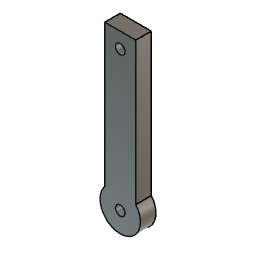
final Assembly (Autodesk Fusion 360 archive; units mm, degrees)
design "link"
Autodesk Fusion 360 part; units mm, degrees
sketch "Sketch1" plane through (0, 0, 0) normal (0, 1, 0) x (1, 0, 0)
  line L0 (0, 0) -> (10, 0)
  line L1 (10, 0) -> (10, 45.8467)
  line L2 (0, 45.8467) -> (0, 0)
  line L3 (0, 0) -> (5, 0)
  circle A0 centre (5, 5) radius 1.55
  circle A1 centre (5, 50) radius 1.55
  arc A2 (10, 45.8467) -> (0, 45.8467) centre (5, 50) ccw
  dimension "d1" = 10
  dimension "d4" = 3.1
  dimension "d5" = 3.1
  dimension "d6" = 13
  constraint horizontal L0
  constraint vertical L1
  constraint vertical L2
  constraint coincident L0.start L2.end
  constraint midpoint L0 L3.end
  constraint concentric A1 A2
  measures "d1" distance of L0.start L0.end
  measures "d4" diameter of A0
  measures "d5" diameter of A1
  measures "d6" diameter of A2
extrude "Extrude1" add sketch "Sketch1" along normal blind 5 contours L0 L1 L2 L3 A2 | A0
extrude "Extrude2" add sketch "Sketch1" along normal blind 10 contours L0 L1 L2 L3 A2 | A0
extrude "Extrude3" add sketch "Sketch1" against normal blind 3 contours L0 L1 L2 L3 A2 | A0
extrude "Extrude4" cut 1 faces at (6.6667, 10, -15.2822) along direction (0, -1, 0) blind 2
extrude "Extrude5" add sketch "Sketch1" against normal blind 8 contours A0
delete_face "DeleteFace1" 1 faces at (6.5423, -4.6667, -4.8457)
sketch "Sketch2" plane through (0, 0, 0) normal (0, 1, 0) x (1, 0, 0)
extrude "Extrude7" cut 1 faces at (6.6667, -3, -15.2822) along direction (0, 1, 0) blind 3
extrude "Extrude8" cut sketch "Sketch1" along normal blind 100 contours A0
extrude "Extrude9" cut 1 faces at (5.0386, 0, -32.7463) along direction (0, 1, 0) blind 3
sketch "Sketch3" plane through (0, 3, 0) normal (0, -1, 0) x (1, 0, 0)
  circle A0 centre (5, -5) radius 1.55
  circle A1 centre (5, -50) radius 1.55
  arc A2 (0, -45.8467) -> (10, -45.8467) centre (5, -50) ccw
  line L0 (10, -45.8467) -> (10, 0)
  line L1 (10, 0) -> (0, 0)
  line L2 (0, 0) -> (0, -45.8467)
extrude "Extrude6" [rolled back] along distance 5 taper angle 0
component "Component" placed x (1, 0, 0) y (0, 1, 0) z (0, 0, 1) at (0, 0, 0)

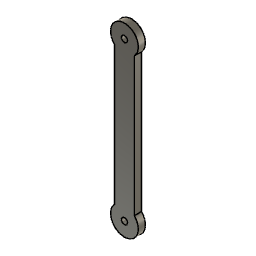
design "new link"
Autodesk Fusion 360 part; units mm, degrees
sketch "Sketch1" plane through (0, 0, 0) normal (0, 1, 0) x (1, 0, 0)
  line L0 (-5, 29.899) -> (-5, -40.101)
  line L1 (5, -40.101) -> (5, 29.899)
  circle A0 centre (0, -45) radius 1.55
  arc A1 (-5, -40.101) -> (5, -40.101) centre (0, -45) ccw
  arc A2 (5, 29.899) -> (-5, 29.899) centre (0, 34.798) ccw
  circle A3 centre (0, 34.798) radius 1.55
  dimension "d3" = 3.1
  dimension "d4" = 14
  dimension "d7" = 70
  dimension "d8" = 7
  dimension "d9" = 3.1
  constraint parallel L0 L1
  constraint concentric A0 A1
  constraint coincident A2.centre A3.centre
  measures "d3" diameter of A0
  measures "d4" diameter of A1
  measures "d7" distance of L1.start L1.end
  measures "d8" radius of A2
  measures "d9" diameter of A3
extrude "Extrude1" add sketch "Sketch1" along normal blind 5
sketch "Sketch2" plane through (0, 0, 0) normal (0, -1, 0) x (1, 0, 0)
  circle A0 centre (0, -34.798) radius 1.55
  circle A1 centre (0, 45) radius 1.55
  arc A2 (-5, -29.899) -> (5, -29.899) centre (0, -34.798) ccw
  line L0 (5, -29.899) -> (5, 40.101)
  arc A3 (5, 40.101) -> (-5, 40.101) centre (0, 45) ccw
  line L1 (-5, 40.101) -> (-5, -29.899)
extrude "Extrude2" cut sketch "Sketch2" against normal blind 1
extrude "Extrude3" cut 1 faces at (-1.6667, 1, 16.7677) along direction (0, 1, 0) blind 0.4

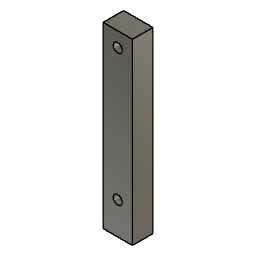
design "link2"
Autodesk Fusion 360 part; units mm, degrees
sketch "Sketch1" plane through (0, 0, 0) normal (0, 1, 0) x (1, 0, 0)
  line L0 (5, 27.5) -> (-5, 27.5)
  line L1 (-5, 27.5) -> (-5, -27.5)
  line L2 (-5, -27.5) -> (5, -27.5)
  line L3 (5, -27.5) -> (5, 27.5)
  line L4 (5, 27.5) -> (-5, -27.5) construction
  line L5 (-5, 27.5) -> (5, -27.5) construction
  line L6 (0, -24.05) -> (0, -22.5)
  circle A0 centre (0, -22.5) radius 1.55
  circle A1 centre (0, 22.5) radius 1.55
  dimension "d1" = 10
  dimension "d2" = 55
  dimension "d4" = 3.1
  constraint horizontal L0
  constraint perpendicular L0 L1
  constraint parallel L0 L2
  constraint parallel L1 L3
  constraint coincident L4 origin
  constraint coincident L5 origin
  constraint perpendicular L2 L6
  constraint coincident L6.end A0.centre
  constraint coincident A0 L6.start
  measures "d1" distance of L1.end L2.end
  measures "d2" distance of L0.end L1.end
  measures "d4" diameter of A0
extrude "Extrude1" add sketch "Sketch1" along normal blind 5
sketch "Sketch2" plane through (0, 0, -27.5) normal (0, 0, -1) x (1, 0, 0)
  line L0 (5, 0) -> (-5, 0)
  line L1 (-5, 0) -> (-5, -5)
  line L2 (-5, -5) -> (5, -5)
  line L3 (5, -5) -> (5, 0)
  circle A0 centre (0, -2.5) radius 1.75
  dimension "d7" = 2.5
  dimension "d8" = 3.5
  measures "d7" distance of origin A0.centre
  measures "d8" diameter of A0
extrude "Extrude2" cut sketch "Sketch2" against normal blind 2 contours A0
extrude "Extrude3" add 1 faces at (3.9167, 2.5, -27.5) along direction (0, 0, -1) blind 6
extrude "Extrude4" add 1 faces at (-0.3896, 1.8511, -25.5) along direction (0, 0, -1) blind 2
extrude "Extrude5" add 1 faces at (-0.0386, 5, -30.3486) along direction (0, 1, 0) blind 1
extrude "Extrude6" add 1 faces at (-0.0386, 0, -30.3486) along direction (0, -1, 0) blind 1
